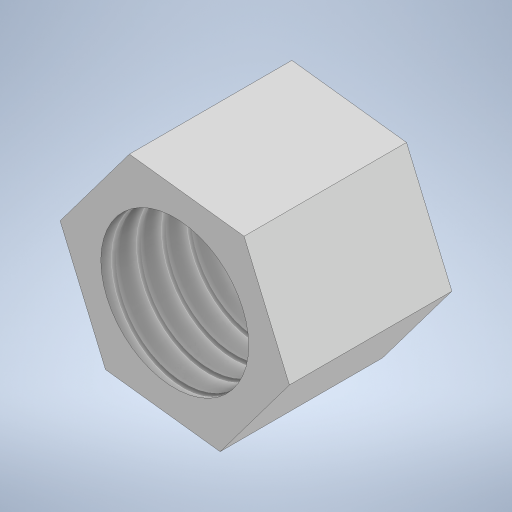
# Autodesk Inventor part: HUDSON-1-108
Saved by Autodesk Inventor 2024.2 (Build 282272000, 272)
## iProperties
Created: 2024-11-02
Part Number: HUDSON-1-108
Material: Generic
Document SubType Name: Modeling
Designer: melim
Density: 1 g/cm^3
Appearance: Default
Author: melim
Autodesk Inventor part; units mm, degrees
ref_plane "YZ Plane" through (0, 0, 0) normal (1, 0, 0) x (0, 1, 0)
ref_plane "XZ Plane" through (0, 0, 0) normal (0, 1, 0) x (-1, 0, 0)
ref_plane "XY Plane" through (0, 0, 0) normal (0, 0, 1) x (1, 0, 0)
sketch "Sketch1" plane through (0, 0, 0) normal (0, 0, 1) x (1, 0, 0)
  line L0 (-5.5426, -7.3901) -> (-9.1713, 1.105)
  line L1 (-9.1713, 1.105) -> (-3.6287, 8.495)
  line L2 (-3.6287, 8.495) -> (5.5426, 7.3901)
  line L3 (5.5426, 7.3901) -> (9.1713, -1.105)
  line L4 (9.1713, -1.105) -> (3.6287, -8.495)
  line L5 (3.6287, -8.495) -> (-5.5426, -7.3901)
  point P0 (0, 0)
  point P1 (0, 0)
  dimension "d0" = 16
  constraints: 12 end point, 1 coincident, 13 other
  measures "d0" distance between parallel lines of L4 L1
extrude "Extrusion1" add sketch "Sketch1" along normal blind 13
sketch "Sketch2" plane through (0, 0, 13) normal (0, 0, 1) x (1, 0, 0)
  point P0 (0, 0)
hole "Hole1" at (0, 0, 13) direction (0, 0, -1) diameter 11.835 depth 9 thread size "M14x2" class "6H" standard "ANSI Metric M Profile"
sketch "Sketch3" plane through (0, 0, 0) normal (0, 0, -1) x (-1, 0, 0)
  point P0 (0, 0)
hole "Hole2" at (0, 0, 0) direction (0, 0, 1) diameter 10 depth 9
body "Solid1"
